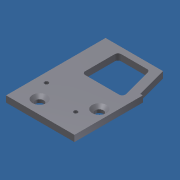
# Autodesk Inventor part: LATERAL-ESQUERDA
Saved by Autodesk Inventor 2012 SP1 (Build 160190100, 190)
## iProperties
Created: 2012-07-23
Part Number: LATERAL-ESQUERDA
Material: Carbon Steel
Document SubType Name: Modeling
Designer: bruno.silveira
Density: 7.87 g/cm^3
Mass: 130.183 g
Surface Area: 88.2317 cm^2
Volume: 16.5417 cm^3
Author: bruno.silveira
Autodesk Inventor part; units mm, degrees
ref_plane "YZ Plane" through (0, 0, 0) normal (1, 0, 0) x (0, 1, 0)
ref_plane "XZ Plane" through (0, 0, 0) normal (0, 1, 0) x (-1, 0, 0)
ref_plane "XY Plane" through (0, 0, 0) normal (0, 0, 1) x (1, 0, 0)
sketch "Sketch1" plane through (0, 0, 0) normal (0, 0, 1) x (1, 0, 0)
  line L0 (0, 0) -> (55, 0)
  line L1 (55, 0) -> (55, 80)
  line L2 (55, 80) -> (0, 80)
  line L3 (0, 80) -> (0, 0)
  dimension "d0" = 55
  dimension "d1" = 80
  constraints: 8 end point, 2 parallel, 1 horizontal, 1 perpendicular
  measures "d0" distance of L0.start L0.end
  measures "d1" distance of L2.end L0.start
extrude "Extrusion1" add sketch "Sketch1" along normal blind 5
sketch "Sketch2" plane through (0, 0, 5) normal (0, 0, 1) x (1, 0, 0)
  line L0 (55, 80) -> (55, 0) projected
  line L1 (0, 80) -> (55, 80) projected
  line L2 (55, 48) -> (53, 48)
  line L3 (53, 48) -> (44.4256, 80)
  line L4 (55, 0) -> (0, 0) projected
  dimension "d4" = 2
  dimension "d5" = 15
  dimension "d38" = 48
  constraints: 4 end point, 2 point on line, 1 parallel
  measures "d4" distance of L2.start L2.end
  measures "d5" angle of L0 L3
  measures "d38" distance between parallel lines of L4 L2
extrude "Extrusion2" cut sketch "Sketch2" against normal blind 5
sketch "Sketch3" plane through (0, 0, 5) normal (0, 0, 1) x (1, 0, 0)
  line L0 (55, 48) -> (53, 48) projected
  line L1 (53, 48) -> (44.4256, 80) projected
  line L2 (0, 80) -> (44.4256, 80) projected
  line L3 (0, 0) -> (0, 80) projected
  line L4 (15, 46) -> (46.289, 46)
  line L5 (38.5184, 75) -> (15, 75)
  line L6 (15, 75) -> (15, 46)
  line L7 (46.289, 46) -> (38.5184, 75)
  dimension "d8" = 29
  dimension "d9" = 15
  dimension "d10" = 5
  dimension "d11" = 7
  constraints: 8 end point, 3 parallel, 1 horizontal
  measures "d8" distance of L5.end L4.start
  measures "d9" distance between parallel lines of L3 L6
  measures "d10" distance between parallel lines of L2 L5
  measures "d11" distance between parallel lines of L1 L7
extrude "Extrusion3" cut sketch "Sketch3" against normal blind 5
fillet "Fillet1" radius 2.5 4 edges at (46.289, 46, 2.5) (15, 46, 2.5) (15, 75, 2.5) (38.5184, 75, 2.5)
sketch "Sketch4" plane through (0, 0, 5) normal (0, 0, 1) x (1, 0, 0)
  line L0 (0, 0) -> (0, 80) projected
  line L1 (55, 0) -> (0, 0) projected
  line L2 (55, 48) -> (55, 0) projected
  point P0 (47, 28)
  point P1 (16, 11)
  dimension "d15" = 16
  dimension "d16" = 11
  dimension "d17" = 28
  dimension "d18" = 8
  measures "d15" distance from line of L0 point (16, 11)
  measures "d16" distance from line of L1 point (16, 11)
  measures "d17" distance from line of L1 point (47, 28)
  measures "d18" distance from line of L2 point (47, 28)
hole "Hole1" at (47, 28, 5) at (16, 11, 5) direction (0, 0, -1) diameter 6.5 depth 5 tip angle 118 countersink diameter 11.5 countersink angle 90
sketch "Sketch5" plane through (0, 0, 0) normal (0, 0, -1) x (-1, 0, 0)
  line L0 (-55, 0) -> (-55, 48) projected
  line L1 (0, 0) -> (-55, 0) projected
  line L2 (0, 80) -> (0, 0) projected
  point P0 (-7.5, 25)
  point P1 (-39.5, 16.5)
  dimension "d26" = 16.5
  dimension "d27" = 15.5
  dimension "d28" = 25
  dimension "d29" = 7.5
  measures "d26" distance from line of L1 point (-39.5, 16.5)
  measures "d27" distance from line of L0 point (-39.5, 16.5)
  measures "d28" distance from line of L1 point (-7.5, 25)
  measures "d29" distance from line of L2 point (-7.5, 25)
hole "Hole2" at (7.5, 25, 0) at (39.5, 16.5, 0) direction (0, 0, 1) diameter 3.175 depth 5 tip angle 118 countersink diameter 4 countersink angle 90
body "Solid1"
